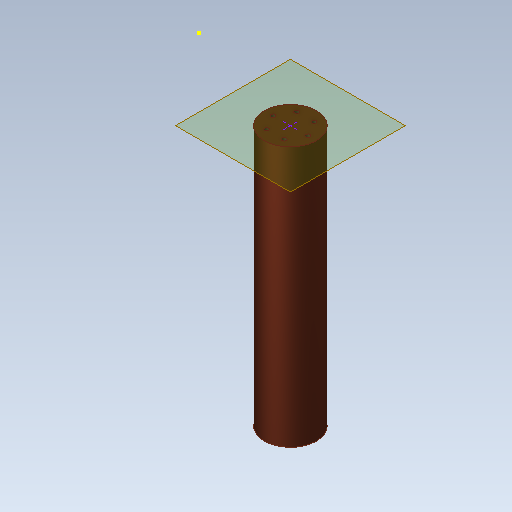
# Autodesk Inventor part: base_stange
Saved by Autodesk Inventor 2020.5 (Build 245400000, 400)
## iProperties
Created: 2018-10-24
Part Number: base_stange
Material: Copper
Document SubType Name: Modeling
Designer: Vi Quint Duong
Density: 8.94 g/cm^3
Appearance: Copper - Satin
Mass: 7552.12 g
Surface Area: 650.03 cm^2
Volume: 844.756 cm^3
Author: Vi Quint Duong
Autodesk Inventor part; units mm, degrees
ref_plane "YZ Plane" through (0, 0, 0) normal (1, 0, 0) x (0, 1, 0)
ref_plane "XZ Plane" through (0, 0, 0) normal (0, 1, 0) x (-1, 0, 0)
ref_plane "XY Plane" through (0, 0, 0) normal (0, 0, 1) x (1, 0, 0)
ref_plane "Work Plane1" through (145.6317, -63.3782, 40.395) normal (0, -1, 0) x (1, 0, 0)
sketch "Sketch1" plane through (145.6317, -63.3782, 40.395) normal (0, -1, 0) x (1, 0, 0)
  circle A0 centre (0, 0) radius 60 projected
  circle A1 centre (0, 0) radius 30
  point P0 (-145.6317, -40.395)
  dimension "d0" = 60
  constraints: 1 centre point, 1 coincident
  measures "d0" diameter of A1
extrude "Extrusion1" add sketch "Sketch1" along normal blind 300 contours A1
sketch "Sketch2" plane through (145.6317, -63.3782, 40.395) normal (0, 1, 0) x (1, 0, 0)
  circle A0 centre (-20, 0) radius 3.3 projected
  circle A1 centre (-10, 17.3205) radius 3.3 projected
  circle A2 centre (10, 17.3205) radius 5.5 projected
  circle A3 centre (10, 17.3205) radius 3.3 projected
  circle A4 centre (20, 0) radius 3.3 projected
  circle A5 centre (10, -17.3205) radius 3.3 projected
  circle A6 centre (-10, -17.3205) radius 3.3 projected
  point P0 (-145.6317, 40.395)
hole "Hole1" at (135.6317, -63.3782, 23.0745) at (155.6317, -63.3782, 23.0745) at (165.6317, -63.3782, 40.395) at (155.6317, -63.3782, 57.7155) at (135.6317, -63.3782, 57.7155) at (125.6317, -63.3782, 40.395) direction (0, -1, 0) diameter 4.917 depth 30 tip angle 118 thread size "M6x1" class "6H" standard "ISO Metric profile"
sketch "Sketch3" plane through (145.6317, -63.3782, 40.395) normal (0, 1, 0) x (1, 0, 0)
  point P0 (-145.6317, 40.395)
  point P1 (0, 0)
body "Solid1"
